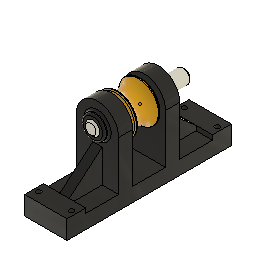
Advance Design 1 v1 (Autodesk Fusion 360 design; units mm, degrees)
Autodesk Fusion 360 part; units mm, degrees
sketch "Sketch1" plane through (0, 0, 0) normal (1, 0, 0) x (0, 1, 0) in component "Base "
  line L0 (-875, 75) -> (875, 75)
  line L1 (875, 75) -> (875, -75)
  line L2 (875, -75) -> (-875, -75)
  line L3 (-875, -75) -> (-875, 75)
  line L4 (175, 75) -> (325, 75)
  line L5 (325, 75) -> (325, 825)
  line L6 (325, 825) -> (175, 825)
  line L7 (175, 825) -> (175, 75)
  line L8 (875, 75) -> (675, 75)
  line L9 (675, 75) -> (675, 125)
  line L10 (675, 125) -> (875, 125)
  line L11 (875, 125) -> (875, 75)
  line L12 (675, 125) -> (325, 425)
  line L13 (-325, 75) -> (-325, 825)
  line L14 (-325, 825) -> (-175, 825)
  line L15 (-175, 75) -> (-325, 75)
  line L16 (-175, 825) -> (-175, 75)
  line L17 (-675, 125) -> (-325, 425)
  line L18 (-675, 75) -> (-675, 125)
  line L19 (-875, 125) -> (-875, 75)
  line L20 (-675, 125) -> (-875, 125)
  dimension "d1" = 1750
  dimension "d2" = 150
  dimension "d3" = 150
  dimension "d4" = 750
  dimension "d5" = 200
  dimension "d6" = 50
  dimension "d7" = 400
  dimension "d8" = 350
  constraint horizontal L0
  constraint perpendicular L0 L1
  constraint parallel L0 L2
  constraint parallel L1 L3
  constraint horizontal L4
  constraint vertical L5
  constraint horizontal L6
  constraint vertical L7
  constraint coincident L0 L4.start
  constraint horizontal L8
  constraint vertical L9
  constraint horizontal L10
  constraint vertical L11
  constraint coincident L5 L12.end
  measures "d1" distance of L1.end L2.end
  measures "d2" distance of L0.end L1.end
  measures "d3" distance of L4.start L4.end
  measures "d4" distance of L4.start L6.end
  measures "d5" distance of L0.end L8.end
  measures "d6" distance of L0.end L10.end
  measures "d7" distance of L5.end L12.end
  measures "d8" distance of L5 L9.end
extrude "Extrude1" add sketch "Sketch1" along normal mid plane 450 contours L0 L18 L19 L20 | L0 L1 L2 L3 L4 L8 L15 | L0 L13 L14 L15 L16 | L0 L8 L9 L10 L11 | L0 L4 L5 L6 L7 makes body 1 in component "Base "
extrude "Extrude2" add sketch "Sketch1" along normal mid plane 100 contours L0 L13 L17 L18 | L0 L5 L9 L12 bodies 1 in component "Base "
fillet "Fillet1" radius 225 4 edges at (-225, -250, 825) (225, -250, 825) (225, 250, 825) (-225, 250, 825) on bodies 1 in component "Base "
sketch "Sketch2" plane through (0, -325, 0) normal (0, -1, 0) x (1, 0, 0) in component "Base "
  arc A0 (225, 600) -> (-225, 600) centre (0, 600) ccw
  line L0 (-225, 600) -> (-225, 75)
  line L1 (-225, 75) -> (-50, 75)
  line L2 (-50, 75) -> (-50, 425)
  line L3 (-50, 425) -> (50, 425)
  line L4 (50, 425) -> (50, 75)
  line L5 (50, 75) -> (225, 75)
  line L6 (225, 75) -> (225, 600)
  circle A1 centre (0, 600) radius 125
  dimension "d15" = 250
  constraint concentric A0 A1
  measures "d15" diameter of A1
extrude "Extrude3" add sketch "Sketch2" along normal blind 50 contours A1 bodies 1 in component "Base "
sketch "Sketch3" plane through (0, -175, 0) normal (0, 1, 0) x (-1, 0, 0) in component "Base "
  arc A0 (225, 600) -> (-225, 600) centre (0, 600) ccw
  line L0 (-225, 600) -> (-225, 75)
  line L1 (-225, 75) -> (225, 75)
  line L2 (225, 75) -> (225, 600)
  circle A1 centre (0, 600) radius 100
  dimension "d18" = 200
  constraint concentric A0 A1
  measures "d18" diameter of A1
extrude "Extrude4" add sketch "Sketch3" along normal blind 20 contours A1 bodies 1 in component "Base "
fillet "Fillet2" radius 20 2 edges at (-116.5409, -375, 554.7981) (-116.5409, -325, 645.2019) on bodies 1 in component "Base "
fillet "Fillet3" radius 10 2 edges at (93.2327, -155, 563.8385) (93.2327, -175, 636.1615) on bodies 1 in component "Base "
hole "Hole1" at (0, -375, 600) direction (0, 1, 0) diameter 150 end through all bodies 1 in component "Base "
mirror "Mirror1" about plane through (0, 0, 0) normal (0, 1, 0) of "Extrude3", "Extrude4", "Fillet2", "Fillet3", "Hole1" in component "Base "
hole "Hole2" at (-175, -775, 125) direction (0, 0, -1) diameter 50 end through all bodies 1 in component "Base "
mirror "Mirror2" about plane through (0, 0, 0) normal (1, 0, 0) of "Hole2" in component "Base "
mirror "Mirror3" about plane through (0, 0, 0) normal (0, 1, 0) of "Hole2", "Mirror2" in component "Base "
sketch "Sketch1 (2)" plane through (0, 0, 0) normal (1, 0, 0) x (0, 1, 0) in component "Roller "
  line L0 (175, 710) -> (175, 825)
  line L1 (175, 75) -> (175, 490)
  line L2 (155, 510) -> (155, 690)
  line L3 (325, 825) -> (325, 745)
  line L4 (325, 455) -> (325, 425)
  line L5 (375, 600) -> (375, 495)
  line L6 (375, 705) -> (375, 600)
  line L7 (-875, 125) -> (-675, 125)
  line L8 (-875, -75) -> (-875, 125)
  line L9 (875, -75) -> (-875, -75)
  line L10 (875, 125) -> (875, -75)
  line L11 (675, 125) -> (875, 125)
  line L12 (-175, 75) -> (175, 75)
  line L13 (-675, 125) -> (-325, 425)
  line L14 (325, 425) -> (675, 125)
  line L15 (-325, 425) -> (-325, 455)
  line L16 (-175, 490) -> (-175, 75)
  line L17 (-325, 745) -> (-325, 825)
  line L18 (-175, 825) -> (-175, 710)
  line L19 (-375, 600) -> (-375, 705)
  line L20 (-375, 495) -> (-375, 600)
  line L21 (-155, 690) -> (-155, 510)
  arc A0 (165, 700) -> (175, 710) centre (165, 710) ccw
  arc A1 (175, 490) -> (165, 500) centre (165, 490) ccw
  arc A2 (165, 700) -> (155, 690) centre (165, 690) ccw
  arc A3 (155, 510) -> (165, 500) centre (165, 510) ccw
  arc A4 (345, 475) -> (325, 455) centre (345, 455) ccw
  arc A5 (325, 745) -> (345, 725) centre (345, 745) ccw
  line L22 (355, 725) -> (345, 725)
  line L23 (355, 475) -> (345, 475)
  arc A6 (355, 475) -> (375, 495) centre (355, 495) ccw
  arc A7 (375, 705) -> (355, 725) centre (355, 705) ccw
  line L24 (-325, 825) -> (-175, 825)
  line L25 (325, 825) -> (175, 825)
  arc A8 (-375, 495) -> (-355, 475) centre (-355, 495) ccw
  arc A9 (-355, 725) -> (-375, 705) centre (-355, 705) ccw
  line L26 (-345, 725) -> (-355, 725)
  line L27 (-345, 475) -> (-355, 475)
  arc A10 (-345, 725) -> (-325, 745) centre (-345, 745) ccw
  arc A11 (-325, 455) -> (-345, 475) centre (-345, 455) ccw
  arc A12 (-155, 690) -> (-165, 700) centre (-165, 690) ccw
  arc A13 (-165, 500) -> (-155, 510) centre (-165, 510) ccw
  arc A14 (-165, 500) -> (-175, 490) centre (-165, 490) ccw
  arc A15 (-175, 710) -> (-165, 700) centre (-165, 710) ccw
  line L28 (-155, 690) -> (-135, 690)
  line L29 (-135, 690) -> (-135, 815)
  line L30 (-135, 815) -> (-115, 815)
  line L31 (0, 75) -> (0, 600) construction
  line L32 (155, 690) -> (135, 690)
  line L33 (135, 690) -> (135, 815)
  line L34 (135, 815) -> (115, 815)
  arc A16 (-115, 815) -> (115, 815) centre (0, 911.3068) ccw
  line L35 (-155, 600) -> (155, 600)
  dimension "d39" = 20
  dimension "d40" = 125
  dimension "d41" = 20
  dimension "d42" = 150
  constraint coincident L21.start A12.start
  constraint perpendicular L21 L28
  constraint perpendicular L28 L29
  constraint perpendicular L29 L30
  constraint midpoint L12 L31.start
  constraint perpendicular L12 L31
  constraint symmetric L21.start L31 L2.end
  constraint symmetric L28.end L31 L32.end
  constraint symmetric L29.end L31 L33.end
  constraint symmetric L30.end L31 L34.end
  constraint midpoint L21 L35.start
  constraint midpoint L2 L35.end
  measures "d39" distance of L21.start L28.end
  measures "d40" distance of L28.end L29.end
  measures "d41" distance of L29.end L30.end
  measures "d42" radius of A16
revolve "Revolve1" add sketch "Sketch1 (2)" angle 360 about axis through (0, -155, 600) along (0, 1, 0) separate body contours L2 L21 L28 L29 L30 L32 L33 L34 A16 L35 makes body 2 in component "Roller "
fillet "Fillet1'" radius 10 8 edges at (-83.9095, -155, 632.5454) (-200.4504, -135, 677.7473) (-200.4504, -115, 677.7473) (-200.4504, 115, 677.7473) (-200.4504, 135, 677.7473) (-83.9095, 155, 632.5454) (-83.9095, -135, 632.5454) (-83.9095, 135, 632.5454) on bodies 2 in component "Roller "
sketch "Sketch2 (2)" plane through (0, 0, 0) normal (0, 0, 1) x (1, 0, 0) in component "Roller "
  circle A0 centre (0, 0) radius 12.5
  dimension "d46" = 25
  constraint coincident A0.centre origin
  measures "d46" diameter of A0
extrude "Extrude1'" cut sketch "Sketch2 (2)" along normal blind 950 bodies 2 in component "Roller "
hole "Hole1'" at (0, -155, 600) direction (0, 1, 0) diameter 150 end through all bodies 2 in component "Roller "
sketch "Sketch1 (3)" plane through (0, -325, 0) normal (0, -1, 0) x (1, 0, 0) in component "Pin"
  arc A0 (225, 600) -> (-225, 600) centre (0, 600) ccw
  line L0 (-225, 600) -> (-225, 75)
  line L1 (-225, 75) -> (-50, 75)
  line L2 (-50, 75) -> (-50, 425)
  line L3 (-50, 425) -> (50, 425)
  line L4 (50, 425) -> (50, 75)
  line L5 (50, 75) -> (225, 75)
  line L6 (225, 75) -> (225, 600)
  circle A1 centre (0, 600) radius 145
  circle A2 centre (0, 600) radius 125
  circle A3 centre (0, 600) radius 75
  dimension "d52" = 250
  dimension "d53" = 150
  constraint concentric A0 A2
  constraint concentric A0 A3
  measures "d52" diameter of A2
  measures "d53" diameter of A3
extrude "Extrude1''" add sketch "Sketch1 (3)" along normal blind 150 and the other way blind 850 separate body contours A3 makes body 3 in component "Pin"
chamfer "Chamfer1" distance 20 angle 45 2 edges at (-69.9246, -475, 572.8788) (-69.9246, 525, 627.1212) on bodies 3 in component "Pin"
component "Base " placed x (1, 0, 0) y (0, 1, 0) z (0, 0, 1) at (0, 0, 0)
component "Roller " placed x (1, 0, 0) y (0, 1, 0) z (0, 0, 1) at (0, 0, 0)
component "Pin" placed x (1, 0, 0) y (0, 1, 0) z (0, 0, 1) at (0, -70, 0)
